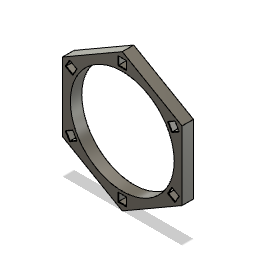
2.5in_hose_coupling v5 (Autodesk Fusion 360 archive; units mm, degrees)
design "2.5_Magnetic_Face"
Autodesk Fusion 360 part; units mm, degrees
sketch "Sketch1" plane through (0, 0, 0) normal (0, 0, 1) x (1, 0, 0)
  circle A0 centre (0, 0) radius 31.75
  line L0 (-36.5295, 21.0903) -> (-36.5295, -21.0903)
  line L1 (-36.5295, -21.0903) -> (0, -42.1806)
  line L2 (0, -42.1806) -> (36.5295, -21.0903)
  line L3 (36.5295, -21.0903) -> (36.5295, 21.0903)
  line L4 (36.5295, 21.0903) -> (0, 42.1806)
  line L5 (0, 42.1806) -> (-36.5295, 21.0903)
  line L6 (-2.375, 33.75) -> (2.375, 33.75)
  line L7 (2.375, 33.75) -> (2.375, 38.5)
  line L8 (2.375, 38.5) -> (-2.375, 38.5)
  line L9 (-2.375, 38.5) -> (-2.375, 33.75)
  line L10 (-2.375, 33.75) -> (2.375, 38.5) construction
  line L11 (2.375, 33.75) -> (-2.375, 38.5) construction
  point P0 (0, 36.125)
  point P1 (0, 31.75)
  dimension "d1" = 63.5
  dimension "d2" = 4.75
  dimension "d3" = 2
  dimension "d4" = 2
  constraint coincident A0.centre origin
  constraint vertical L4.end A0.centre
  constraint horizontal L6
  constraint perpendicular L6 L7
  constraint parallel L6 L8
  constraint parallel L7 L9
  constraint coincident L10 P0
  constraint coincident L11 P0
  constraint equal L7 L8
  constraint vertical A0.centre P0
  constraint coincident A0 P1
  measures "d1" diameter of A0
  measures "d2" distance of L6 L8
  measures "d3" distance of L5 L8.end
  measures "d4" distance of L6 P1
extrude "Extrude1" add sketch "Sketch1" along normal blind 6 contours L0 L1 L2 L3 L4 L5 | L6 L7 L8 L9
extrude "Extrude2" add sketch "Sketch1" against normal blind 1 contours L0 L1 L2 L3 L4 L5 | L6 L7 L8 L9
extrude "Extrude3" cut sketch "Sketch1" along normal blind 33.02 contours L6 L7 L8 L9
sketch "Sketch2" plane through (0, 0, 6) normal (0, 0, 1) x (1, 0, 0)
  line L0 (-2.375, 38.5) -> (2.375, 38.5)
  line L1 (2.375, 38.5) -> (2.375, 33.75)
  line L2 (2.375, 33.75) -> (-2.375, 33.75)
  line L3 (-2.375, 33.75) -> (-2.375, 38.5)
  circle A0 centre (0, 0) radius 31.75
  line L4 (0, 42.1806) -> (-36.5295, 21.0903)
  line L5 (-36.5295, 21.0903) -> (-36.5295, -21.0903)
  line L6 (-36.5295, -21.0903) -> (0, -42.1806)
  line L7 (0, -42.1806) -> (36.5295, -21.0903)
  line L8 (36.5295, -21.0903) -> (36.5295, 21.0903)
  line L9 (36.5295, 21.0903) -> (0, 42.1806)
  line L10 (-8.9538, 50.7426) -> (10.16, 50.7426)
  line L11 (10.16, 50.7426) -> (10.16, 22.86)
  line L12 (10.16, 22.86) -> (-8.9538, 22.86)
  line L13 (-8.9538, 22.86) -> (-8.9538, 50.7426)
  constraint horizontal L10
  constraint vertical L11
  constraint horizontal L12
  constraint vertical L13
extrude "Extrude4" [suppressed]
chamfer "Chamfer1" distance 0.25 angle 45 4 edges at (-2.375, 36.125, 6) (0, 33.75, 6) (2.375, 36.125, 6) (0, 38.5, 6) measured on face at (34.9363, 0, 6) measured on face at (34.9363, 0, 6) measured on face at (34.9363, 0, 6) measured on face at (34.9363, 0, 6)
sketch "Sketch3" plane through (0, 0, 0) normal (0, 0, 1) x (1, 0, 0)
  line L0 (-2.375, 38.5) -> (-2.375, 33.75)
  line L1 (-2.375, 33.75) -> (2.375, 33.75)
  line L2 (2.375, 33.75) -> (2.375, 38.5)
  line L3 (2.375, 38.5) -> (-2.375, 38.5)
  line L4 (2.375, 38.5) -> (-2.375, 33.75)
  point P0 (0, 36.125)
  constraint coincident L2.end L3.start
  constraint coincident L0.end L1.start
  constraint midpoint L4 P0
pattern_circular "C-Pattern1" count 6 over 360 about axis through (0, 0, 1.75) along (0, 0, 1) of "Extrude3", "Chamfer1"
